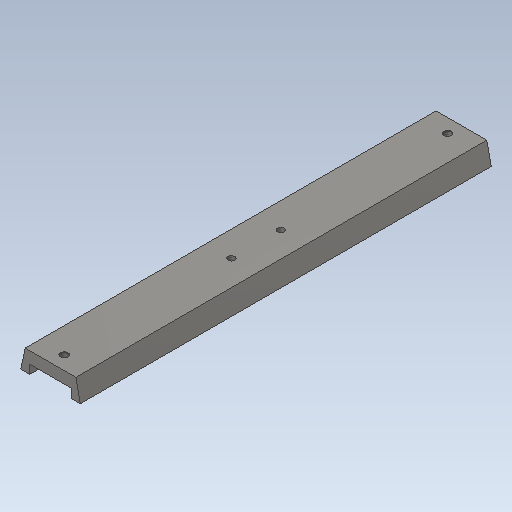
# Autodesk Inventor part: szyna
Saved by Autodesk Inventor 2020 (Build 240168000, 168)
## iProperties
Created: 2019-06-01
Part Number: szyna
Material: Stainless Steel
Document SubType Name: Modeling
Designer: Esterka
Density: 8 g/cm^3
Appearance: Semi-Polished
Author: Esterka
Autodesk Inventor part; units mm, degrees
ref_plane "YZ Plane" through (0, 0, 0) normal (1, 0, 0) x (0, 1, 0)
ref_plane "XZ Plane" through (0, 0, 0) normal (0, 1, 0) x (-1, 0, 0)
ref_plane "XY Plane" through (0, 0, 0) normal (0, 0, 1) x (1, 0, 0)
sketch "Sketch1" plane through (0, 0, 0) normal (0, 0, 1) x (1, 0, 0)
  line L0 (-3.981, 7.2547) -> (33.019, 7.2547)
  line L1 (33.019, 7.2547) -> (36.269, -7.7453)
  line L2 (-7.231, -7.7453) -> (-3.981, 7.2547)
  line L3 (-0.731, -1.2453) -> (29.769, -1.2453)
  line L4 (29.769, -1.2453) -> (29.769, -7.7453)
  line L5 (-0.731, -1.2453) -> (-0.731, -7.7453)
  line L6 (36.269, -7.7453) -> (29.769, -7.7453)
  line L7 (-0.731, -7.7453) -> (-7.231, -7.7453)
  point P0 (0, 0)
  dimension "d0" = 37
  dimension "d1" = 43.5
  dimension "d4" = 30.5
  constraints: 16 end point, 2 horizontal, 2 parallel, 2 perpendicular, 1 vertical
  measures "d0" distance of L0.start L0.end
  measures "d1" distance of L1.end L2.start
  measures "d4" distance of L3.start L3.end
extrude "Extrusion1" add sketch "Sketch1" along normal blind 300
sketch "Sketch2" plane through (-3.981, 7.2547, 0) normal (0, 1, 0) x (1, 0, 0)
  line L0 (37, -300) -> (0, -300) projected
  line L1 (0, 0) -> (37, 0) projected
  point P0 (3.981, 0)
  point P1 (18.5, -10)
  point P2 (18.5, -132)
  point P3 (18.5, -168)
  point P4 (18.5, -290)
  dimension "d9" = 10
  dimension "d10" = 10
  dimension "d11" = 36
  measures "d9" distance from line of L0 point (18.5, -290)
  measures "d10" distance from line of L1 point (18.5, -10)
  measures "d11" distance of point (18.5, -132) point (18.5, -168)
hole "Hole1" at (14.519, 7.2547, 10) at (14.519, 7.2547, 132) at (14.519, 7.2547, 168) at (14.519, 7.2547, 290) direction (0, -1, 0) diameter 4.978 end through all thread size "1/4-20 UNC" class "2B" standard "ANSI Unified Screw Threads"
chamfer "Chamfer1" distance 0.3 angle 45 4 edges at (14.519, 7.2547, 287.511) (14.519, 7.2547, 7.511) (14.519, -1.2453, 129.511) (14.519, -1.2453, 165.511)
body "Solid1"
